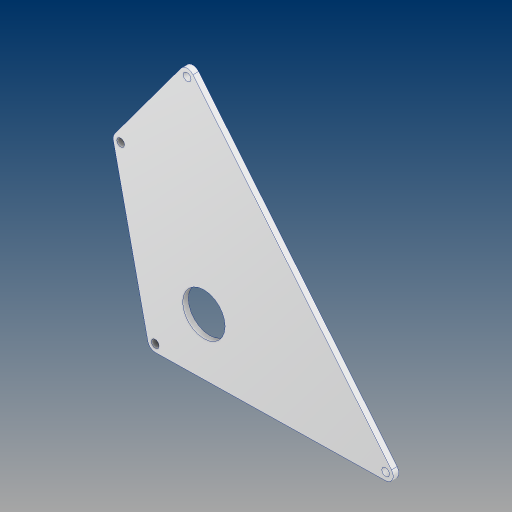
# Autodesk Inventor part: SHOT_1_015_PivotCover
Saved by Autodesk Inventor 2024.3 (Build 283343000, 343)
## iProperties
Created: 2024-08-09
Part Number: SHOT_1_015_PivotCover
Material: Aluminum 6061
Document SubType Name: Modeling
Designer: Kenji
Density: 2.7 g/cm^3
Appearance: Aluminum - Flat
Author: Kenji
Autodesk Inventor part; units mm, degrees
ref_plane "YZ Plane" through (0, 0, 0) normal (1, 0, 0) x (0, 1, 0)
ref_plane "XZ Plane" through (0, 0, 0) normal (0, 1, 0) x (-1, 0, 0)
ref_plane "XY Plane" through (0, 0, 0) normal (0, 0, 1) x (1, 0, 0)
sketch "Sketch2" plane through (0, 0, 0) normal (0, 0, 1) x (1, 0, 0)
  line L0 (0, 0) -> (264.075, 76.1785) construction
  circle A0 centre (264.075, 76.1785) radius 3.2512
  line L1 (0, 0) -> (41.9951, 204.3053) construction
  circle A1 centre (41.9951, 204.3053) radius 3.2512
  line L2 (0, 0) -> (97.7, 279.7575) construction
  circle A2 centre (97.7, 279.7575) radius 3.2512
  line L3 (0, 0) -> (70.949, 72.7241) construction
  circle A3 centre (70.949, 72.7241) radius 3.2512
  circle A4 centre (0, 0) radius 142.24 construction
  circle A5 centre (111.7447, 114.5405) radius 17.78
  circle A6 centre (111.7447, 114.5405) radius 30 construction
  circle A7 centre (97.7, 279.7575) radius 6.35 construction
  circle A8 centre (41.9951, 204.3053) radius 6.35 construction
  circle A9 centre (70.949, 72.7241) radius 6.35 construction
  circle A10 centre (264.075, 76.1785) radius 6.35 construction
  line L4 (102.6169, 283.7758) -> (268.9919, 80.1968)
  line L5 (71.0626, 66.3751) -> (264.1886, 69.8295)
  line L6 (64.7474, 71.3595) -> (35.7934, 202.9407)
  line L7 (36.8865, 208.0769) -> (92.5914, 283.5291)
  arc A11 (36.8865, 208.0769) -> (35.7934, 202.9407) centre (41.9951, 204.3053) ccw
  arc A12 (102.6169, 283.7758) -> (92.5914, 283.5291) centre (97.7, 279.7575) ccw
  arc A13 (264.1886, 69.8295) -> (268.9919, 80.1968) centre (264.075, 76.1785) ccw
  arc A14 (64.7474, 71.3595) -> (71.0626, 66.3751) centre (70.949, 72.7241) ccw
  dimension "d63" = 6.5024
  dimension "d64" = 274.8432
  dimension "d65" = 76.1785
  dimension "d66" = 208.5767
  dimension "d67" = 6.5024
  dimension "d68" = 204.3053
  dimension "d69" = 6.5024
  dimension "d70" = 296.3268
  dimension "d71" = 279.7575
  dimension "d72" = 101.6
  dimension "d73" = 6.5024
  dimension "d74" = 72.7241
  dimension "d75" = 284.48
  dimension "d76" = 35.56
  dimension "d77" = 60
  dimension "d78" = 12.7
  dimension "d79" = 12.7
  dimension "d80" = 12.7
  dimension "d81" = 12.7
  constraints: 17 point on circle, 16 end point, 15 centre point, 11 tangent, 10 coincident, 3 concentric, 1 point on line, 1 other
  measures "d63" diameter of A0
  measures "d64" distance of L0.start L0.end
  measures "d65" vertical distance of L0.start L0.end
  measures "d66" distance of L0.start L1.end
  measures "d67" diameter of A1
  measures "d68" vertical distance of L0.start L1.end
  measures "d69" diameter of A2
  measures "d70" distance of L0.start L2.end
  measures "d71" vertical distance of L0.start L2.end
  measures "d72" distance of L0.start L3.end
  measures "d73" diameter of A3
  measures "d74" vertical distance of L0.start L3.end
  measures "d75" diameter of A4
  measures "d76" diameter of A5
  measures "d77" diameter of A6
  measures "d78" diameter of A7
  measures "d79" diameter of A8
  measures "d80" diameter of A9
  measures "d81" diameter of A10
extrude "Extrusion2" add sketch "Sketch2" along normal blind 4.7625
body "Solid2"
